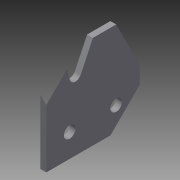
# Autodesk Inventor part: pickup arm tab with hook
Saved by Autodesk Inventor 2015 SP1 (Build 190203100, 203)
## iProperties
Created: 2015-02-05
Part Number: pickup arm tab with hook
Material: Generic
Document SubType Name: Modeling
Designer: Admin
Density: 1 g/cm^3
Appearance: Default
Author: Admin
Autodesk Inventor part; units mm, degrees
ref_plane "YZ Plane" through (0, 0, 0) normal (1, 0, 0) x (0, 1, 0)
ref_plane "XZ Plane" through (0, 0, 0) normal (0, 1, 0) x (-1, 0, 0)
ref_plane "XY Plane" through (0, 0, 0) normal (0, 0, 1) x (1, 0, 0)
sketch "Sketch1" plane through (0, 0, 0) normal (1, 0, 0) x (0, 1, 0)
  line L0 (0, 0) -> (50.8, 0) construction
  line L1 (50.8, 0) -> (50.8, -50.8) construction
  line L2 (50.8, -50.8) -> (0, -50.8) construction
  line L3 (0, -50.8) -> (0, 0) construction
  line L4 (0, 0) -> (50.8, 0)
  line L5 (50.8, 0) -> (50.8, -9.525)
  line L6 (0, 0) -> (0, -50.8)
  line L7 (50.8, -25.4) -> (50.8, -38.1)
  line L8 (50.8, -38.1) -> (25.4, -50.8)
  line L9 (25.4, -50.8) -> (0, -50.8)
  circle A0 centre (38.1, -15.875) radius 3.175 construction
  line L10 (50.8, -9.525) -> (37.351, -12.7896)
  line L11 (50.8, -25.4) -> (36.7415, -18.7447)
  arc A1 (37.351, -12.7896) -> (36.7415, -18.7447) centre (38.1, -15.875) ccw
  dimension "d0" = 50.8
  dimension "d1" = 50.8
  dimension "d2" = 9.525
  dimension "d3" = 12.7
  dimension "d6" = 6.35
  dimension "d7" = 12.7
  dimension "d8" = 15.875
  dimension "d22" = 25.4
  dimension "d23" = 12.7
  constraints: 24 end point, 4 point on circle, 4 tangent, 3 equal length, 2 centre point, 2 horizontal, 2 midpoint, 2 point on line, 1 perpendicular, 1 vertical
  measures "d0" distance of L1.end L2.end
  measures "d1" distance of L0.end L1.end
  measures "d2" distance of L0.end L5.end
  measures "d3" distance of L7.start L7.end
  measures "d6" diameter of A0
  measures "d7" distance from line of A0.centre L1
  measures "d8" distance from line of L0 A0.centre
  measures "d22" distance of L8.end L2.end
  measures "d23" distance from line of L7.end L2
extrude "Extrusion1" add sketch "Sketch1" along normal blind 3.175
sketch "Sketch2" plane through (3.175, 0, 0) normal (1, 0, 0) x (0, 0, -1)
  line L0 (0, 50.8) -> (0, 0) projected
  line L1 (0, 0) -> (50.8, 0) projected
  point P0 (12.7, 12.7)
  point P1 (38.1, 12.7)
  dimension "d11" = 12.7
  dimension "d12" = 12.7
  dimension "d13" = 12.7
  dimension "d14" = 38.1
  measures "d11" distance from line of L1 point (12.7, 12.7)
  measures "d12" distance from line of L0 point (12.7, 12.7)
  measures "d13" distance from line of L1 point (38.1, 12.7)
  measures "d14" distance from line of L0 point (38.1, 12.7)
hole "Hole1" at (3.175, 12.7, -12.7) at (3.175, 12.7, -38.1) direction (-1, 0, 0) diameter 6.35 end through all
body "Solid1"
